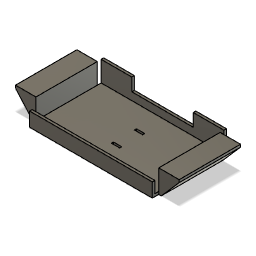
Color Sensor Mount v1 (Autodesk Fusion 360 design; units mm, degrees)
Autodesk Fusion 360 part; units mm, degrees
sketch "Sketch4" plane through (0, 0, 0) normal (0, 1, 0) x (1, 0, 0)
  line L0 (0, 0) -> (152.4, 0)
  line L1 (152.4, 0) -> (152.4, 85.725)
  line L2 (152.4, 85.725) -> (0, 85.725)
  line L3 (0, 85.725) -> (0, 0)
  dimension "d16" = 152.4
  dimension "d17" = 85.725
  constraint coincident L0.start L3.end
  constraint horizontal L0
  constraint perpendicular L0 L1
  constraint perpendicular L1 L2
  constraint perpendicular L2 L3
  measures "d16" distance of L0.start L0.end
  measures "d17" distance of L0.end L1.end
extrude "Extrude4" add sketch "Sketch4" along normal blind 3.175
sketch "Sketch5" plane through (0, 0, 0) normal (0, 0, 1) x (1, 0, 0)
  line L0 (0, 0) -> (152.4, 0)
  line L1 (152.4, 0) -> (152.4, 3.175)
  line L2 (152.4, 3.175) -> (0, 3.175)
  line L3 (0, 3.175) -> (0, 0)
  line L4 (0, 3.175) -> (152.4, 3.175)
  line L5 (0, 0) -> (152.4, 0)
  line L6 (0, 0) -> (0, 3.175)
  line L7 (152.4, 0) -> (152.4, 3.175)
  line L8 (152.4, 0) -> (152.4, 17.4625)
  line L9 (0, 0) -> (0, 17.4625)
  line L10 (0, 17.4625) -> (152.4, 17.4625)
  dimension "d20" = 17.4625
  dimension "d21" = 17.4625
  constraint coincident L0.end L1.start
  constraint perpendicular L4 L8
  constraint coincident L0.start L3.end
  constraint perpendicular L4 L9
  measures "d20" distance of L0.end L8.end
  measures "d21" distance of L0.start L9.end
extrude "Extrude5" add sketch "Sketch5" along normal blind 3.175
sketch "Sketch6" plane through (0, 0, -85.725) normal (0, 0, -1) x (-1, 0, 0)
  line L0 (-152.4, 0) -> (0, 0)
  line L1 (0, 0) -> (0, 3.175)
  line L2 (0, 3.175) -> (-152.4, 3.175)
  line L3 (-152.4, 3.175) -> (-152.4, 0)
  line L4 (-152.4, 3.175) -> (0, 3.175)
  line L5 (-152.4, 0) -> (-152.4, 3.175)
  line L6 (-152.4, 0) -> (0, 0)
  line L7 (0, 0) -> (0, 3.175)
  line L8 (0, 0) -> (0, 28.575)
  line L9 (0, 28.575) -> (-38.1, 28.575)
  line L10 (-38.1, 28.575) -> (-38.1, 12.7)
  line L11 (-38.1, 12.7) -> (-114.3, 12.7)
  line L12 (-114.3, 12.7) -> (-114.3, 28.575)
  line L13 (-114.3, 28.575) -> (-152.4, 28.575)
  line L14 (-152.4, 28.575) -> (-152.4, 0)
  dimension "d24" = 28.575
  dimension "d25" = 38.1
  dimension "d26" = 15.875
  dimension "d27" = 76.2
  dimension "d28" = 15.875
  dimension "d29" = 38.1
  constraint coincident L0.end L1.start
  constraint perpendicular L6 L8
  constraint perpendicular L8 L9
  constraint perpendicular L9 L10
  constraint perpendicular L10 L11
  constraint perpendicular L11 L12
  constraint perpendicular L12 L13
  constraint coincident L0.start L3.end
  measures "d24" distance of L0.end L8.end
  measures "d25" distance of L8.end L9.end
  measures "d26" distance of L9.end L10.end
  measures "d27" distance of L10.end L11.end
  measures "d28" distance of L11.end L12.end
  measures "d29" distance of L12.end L13.end
extrude "Extrude6" add sketch "Sketch6" along normal blind 3.175
sketch "Sketch7" plane through (0, 0, 0) normal (-1, 0, 0) x (0, 0, 1)
  line L0 (-88.9, 0) -> (3.175, 0)
  line L1 (3.175, 0) -> (3.175, 17.4625)
  line L2 (3.175, 17.4625) -> (0, 17.4625)
  line L3 (0, 17.4625) -> (0, 3.175)
  line L4 (0, 3.175) -> (-85.725, 3.175)
  line L5 (-85.725, 3.175) -> (-85.725, 28.575)
  line L6 (-85.725, 28.575) -> (-88.9, 28.575)
  line L7 (-88.9, 28.575) -> (-88.9, 0)
  line L8 (-85.725, 3.175) -> (-85.725, 28.575)
  line L9 (-85.725, 28.575) -> (-88.9, 28.575)
  line L10 (-88.9, 0) -> (-88.9, 28.575)
  line L11 (-85.725, 3.175) -> (0, 3.175)
  line L12 (0, 3.175) -> (0, 17.4625)
  line L13 (0, 17.4625) -> (3.175, 17.4625)
  line L14 (3.175, 17.4625) -> (3.175, 0)
  line L15 (-88.9, 0) -> (3.175, 0)
  line L16 (-85.725, 3.175) -> (-80.9625, 3.175) construction
  line L17 (0, 3.175) -> (-4.7625, 3.175) construction
  line L18 (-80.9625, 0) -> (-80.9625, 28.575)
  line L19 (-4.7625, 0) -> (-4.7625, 28.575)
  line L20 (-80.9625, 28.575) -> (-4.7625, 28.575)
  dimension "d35" = 4.7625
  dimension "d36" = 4.7625
  dimension "d37" = 28.575
  dimension "d38" = 28.575
  dimension "d39" = 76.2
  constraint coincident L4.end L5.start
  constraint perpendicular L5 L16
  constraint coincident L3.end L4.start
  constraint perpendicular L12 L17
  constraint coincident L15 L18.start
  constraint perpendicular L16 L18
  constraint coincident L15 L19.start
  constraint perpendicular L11 L19
  constraint perpendicular L18 L20
  measures "d35" distance of L4.end L16.end
  measures "d36" distance of L3.end L17.end
  measures "d37" distance of L18.start L18.end
  measures "d38" distance of L19.start L19.end
  measures "d39" distance of L18.end L19.end
extrude "Extrude7" add sketch "Sketch7" along normal blind 3.175 contours L0 L4 L11 L15 L18 L19 | L4 L11 L18 L19 L20
sketch "Sketch8" plane through (0, 28.575, 0) normal (0, 1, 0) x (-1, 0, 0)
  line L0 (0, -4.7625) -> (0, -80.9625)
  line L1 (0, -80.9625) -> (3.175, -80.9625)
  line L2 (3.175, -80.9625) -> (3.175, -4.7625)
  line L3 (3.175, -4.7625) -> (0, -4.7625)
  line L4 (0, -80.9625) -> (3.175, -80.9625)
  line L5 (0, -80.9625) -> (0, -4.7625)
  line L6 (3.175, -4.7625) -> (3.175, -80.9625)
  line L7 (0, -4.7625) -> (3.175, -4.7625)
  line L8 (0, -4.7625) -> (25.4, -4.7625)
  line L9 (0, -80.9625) -> (25.4, -80.9625)
  line L10 (25.4, -80.9625) -> (25.4, -4.7625)
  dimension "d42" = 25.4
  dimension "d43" = 25.4
  dimension "d44" = 76.2
  constraint coincident L0.start L3.end
  constraint perpendicular L5 L8
  constraint coincident L0.end L1.start
  constraint perpendicular L5 L9
  constraint perpendicular L8 L10
  measures "d42" distance of L0.start L8.end
  measures "d43" distance of L0.end L9.end
  measures "d44" distance of L9.end L8.end
extrude "Extrude9" add sketch "Sketch8" against normal blind 3.175 contours L2 L6 L8 L9 L10
ref_plane "WorkPlane1" through (76.2, 14.2875, -42.8625) normal (1, 0, 0) x (0, 0, -1)
mirror "Mirror1" about plane through (76.2, 14.2875, -42.8625) normal (1, 0, 0) of "Extrude7"
mirror "Mirror3" about plane through (76.2, 14.2875, -42.8625) normal (1, 0, 0) of "Extrude9"
sketch "Sketch9" plane through (0, 0, -80.9625) normal (0, 0, -1) x (-1, 0, 0)
  line L0 (-152.4, 0) -> (-152.4, 3.175)
  line L1 (-152.4, 3.175) -> (-152.4, 28.575)
  line L2 (-152.4, 28.575) -> (-177.8, 28.575)
  line L3 (-177.8, 28.575) -> (-177.8, 25.4)
  line L4 (-177.8, 25.4) -> (-155.575, 25.4)
  line L5 (-155.575, 25.4) -> (-155.575, 0)
  line L6 (-155.575, 0) -> (-152.4, 0)
  line L7 (-177.8, 25.4) -> (-155.575, 0)
  constraint coincident L3.end L4.start
  constraint coincident L5.end L6.start
extrude "Extrude10" add sketch "Sketch9" against normal up to surface (76.2 mm away) contours L4 L5 L7
mirror "Mirror4" about plane through (76.2, 14.2875, -42.8625) normal (1, 0, 0) of "Extrude10"
sketch "Sketch10" plane through (0, 3.175, 0) normal (0, 1, 0) x (-1, 0, 0)
  line L0 (0, -85.725) -> (0, -80.9625)
  line L1 (0, -80.9625) -> (0, -4.7625)
  line L2 (0, -4.7625) -> (0, 0)
  line L3 (0, 0) -> (-152.4, 0)
  line L4 (-152.4, 0) -> (-152.4, -4.7625)
  line L5 (-152.4, -4.7625) -> (-152.4, -80.9625)
  line L6 (-152.4, -80.9625) -> (-152.4, -85.725)
  line L7 (-152.4, -85.725) -> (0, -85.725)
  line L8 (0, -80.9625) -> (0, -4.7625)
  line L9 (-152.4, -85.725) -> (0, -85.725)
  line L10 (0, -85.725) -> (0, -80.9625)
  line L11 (0, -4.7625) -> (0, 0)
  line L12 (0, 0) -> (-152.4, 0)
  line L13 (-152.4, -4.7625) -> (-152.4, -80.9625)
  line L14 (-152.4, -80.9625) -> (-152.4, -85.725)
  line L15 (-152.4, 0) -> (-152.4, -4.7625)
  line L16 (0, -85.725) -> (-152.4, 0) construction
  line L17 (-152.4, -85.725) -> (0, 0) construction
  line L18 (-76.2, -42.8625) -> (-88.2955, -42.8625) construction
  line L19 (-76.2, -42.8625) -> (-64.1096, -42.8625) construction
  line L20 (-64.1096, -42.8625) -> (-64.1096, -58.3692) construction
  line L21 (-64.1096, -42.8625) -> (-64.1096, -27.3558) construction
  line L22 (-64.1096, -58.3692) -> (-88.2904, -58.3692) construction
  line L23 (-64.1096, -27.3558) -> (-88.2904, -27.3558) construction
  line L24 (-88.2904, -58.3692) -> (-88.2904, -27.3558) construction
  line L25 (-64.1096, -58.3692) -> (-71.12, -58.3692) construction
  line L26 (-88.2904, -58.3692) -> (-81.28, -58.3692) construction
  line L27 (-64.1096, -27.3558) -> (-71.12, -27.3558) construction
  line L28 (-71.12, -58.3692) -> (-71.12, -55.8292)
  line L29 (-71.12, -55.8292) -> (-81.28, -55.8292)
  line L30 (-81.28, -55.8292) -> (-81.28, -58.3692)
  line L31 (-71.12, -58.3692) -> (-81.28, -58.3692)
  line L32 (-71.12, -27.3558) -> (-71.12, -29.8958)
  line L33 (-71.12, -29.8958) -> (-81.28, -29.8958)
  line L34 (-81.28, -29.8958) -> (-81.28, -27.3558)
  line L35 (-64.1096, -27.3558) -> (-88.2904, -27.3558) construction
  line L36 (-71.12, -27.3558) -> (-81.28, -27.3558)
  point P0 (-152.4, -85.725)
  dimension "d61" = 15.5067
  dimension "d62" = 15.5067
  dimension "d63" = 24.1808
  dimension "d64" = 7.0104
  dimension "d65" = 7.0104
  dimension "d66" = 2.54
  constraint coincident L0.start L7.end
  constraint coincident L3.end L4.start
  constraint coincident P0 L6.end
  constraint coincident L2.end L3.start
  constraint midpoint L17 L18.start
  constraint perpendicular L8 L18
  constraint parallel L18 L19
  constraint perpendicular L19 L20
  constraint perpendicular L19 L21
  constraint perpendicular L20 L22
  constraint perpendicular L21 L23
  constraint perpendicular L23 L24
  constraint coincident L22 L25.end
  constraint perpendicular L24 L26
  constraint symmetric L19 L20.end L21.end
  constraint symmetric L19 L25.end L27.end
  constraint perpendicular L22 L28
  constraint perpendicular L28 L29
  constraint perpendicular L26 L30
  constraint symmetric L19 L22.end L23.end
  constraint symmetric L19 L26.end L34.end
  constraint symmetric L19 L28.end L32.end
  constraint symmetric L19 L29.end L33.end
  measures "d61" distance of L19.end L20.end
  measures "d62" distance of L19.end L21.end
  measures "d63" distance of L20.end L22.end
  measures "d64" distance of L20.end L25.end
  measures "d65" distance of L22.end L26.end
  measures "d66" distance of L25.end L28.end
extrude "Extrude11" cut sketch "Sketch10" against normal blind 14.7066 contours L28 L29 L30 L31 | L32 L33 L34 L36
equation "d16 = 6\""
equation "d27 = 3\""
equation "d39 = 3\""
equation "d42 = 1\""
equation "d43 = 1\""
equation "d44 = 3\""
equation "d63 = ( 0.476 in + 0.476 in )"
